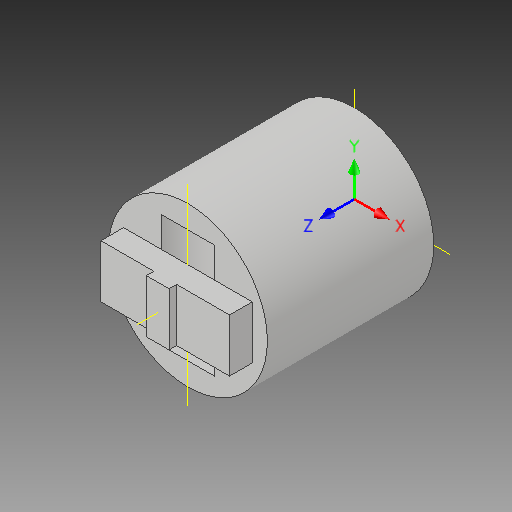
# Autodesk Inventor part: link_1
Saved by Autodesk Inventor 2019 (Build 230136000, 136)
## iProperties
Created: 2020-08-30
Part Number: link_1
Material: Generic
Document SubType Name: Modeling
Designer: Daniel
Density: 1 g/cm^3
Appearance: Default
Author: Daniel
Autodesk Inventor part; units mm, degrees
ref_plane "YZ Plane" through (0, 0, 0) normal (1, 0, 0) x (0, 1, 0)
ref_plane "XZ Plane" through (0, 0, 0) normal (0, 1, 0) x (-1, 0, 0)
ref_plane "XY Plane" through (0, 0, 0) normal (0, 0, 1) x (1, 0, 0)
sketch "Sketch1" plane through (0, 0, 0) normal (0, 0, 1) x (1, 0, 0)
  circle A0 centre (0, 0) radius 84
  dimension "d0" = 168
  constraints: 1 centre point, 1 coincident
  measures "d0" diameter of A0
extrude "Extrusion1" add sketch "Sketch1" along normal blind 176
sketch "Sketch2" plane through (0, 0, 0) normal (0, 1, 0) x (-1, 0, 0)
  line L0 (84, 176) -> (-84, 176) projected
  circle A0 centre (0, 176) radius 28
  point P0 (0, 0)
  dimension "d3" = 56
  constraints: 1 centre point, 1 midpoint
  measures "d3" diameter of A0
extrude "Extrusion2" cut sketch "Sketch2" along normal mid plane 120
sketch "Sketch4" plane through (0, 0, 176) normal (0, 0, 1) x (1, 0, 0)
  line L0 (68, -28) -> (-68, -28)
  line L1 (-68, -28) -> (-68, 28)
  line L2 (-68, 28) -> (68, 28)
  line L3 (68, 28) -> (68, -28)
  line L4 (68, -28) -> (-68, 28) construction
  line L5 (-68, -28) -> (68, 28) construction
  circle A0 centre (0, 0) radius 84 projected
  dimension "d7" = 56
  dimension "d8" = 16
  constraints: 12 end point, 2 midpoint, 2 parallel, 1 horizontal, 1 perpendicular
  measures "d7" distance between parallel lines of L2 L0
  measures "d8" distance edge to line of A0 L1
extrude "Extrusion3" add sketch "Sketch4" along normal blind 24 contours L0 L1 L2 L3
sketch "Sketch5" plane through (0, 0, 200) normal (0, 0, 1) x (1, 0, 0)
  line L0 (28, -28) -> (-28, -28) projected
  line L1 (-12, 28) -> (12, 28)
  line L2 (12, 28) -> (12, -28)
  line L3 (12, -28) -> (-12, -28)
  line L4 (-12, -28) -> (-12, 28)
  line L5 (-12, 28) -> (12, -28) construction
  line L6 (12, 28) -> (-12, -28) construction
  point P0 (0, 0)
  dimension "d11" = 24
  constraints: 12 end point, 2 midpoint, 2 parallel, 1 horizontal, 1 perpendicular, 1 point on line
  measures "d11" distance between parallel lines of L4 L2
extrude "Extrusion4" add sketch "Sketch5" along normal blind 8
body "Solid1"
